clamp for 20mm (Autodesk Fusion 360 design; units mm, degrees)
Autodesk Fusion 360 part; units mm, degrees
note: some values were not read from the file. Set by a fixed rule: which sketch regions a step uses.
sketch "Sketch1" plane through (0, 0, 0) normal (0, 1, 0) x (1, 0, 0)
  line L0 (0, 0) -> (40, 0)
  line L1 (40, 0) -> (40, -16)
  line L2 (40, -16) -> (0, -16)
  line L3 (0, -16) -> (0, 0)
  line L4 (0, -16) -> (40, -16)
  line L5 (40, -16) -> (40, -20)
  line L6 (40, -20) -> (0, -20)
  line L7 (0, -20) -> (0, -16)
  dimension "d1" = 16
  dimension "d2" = 40
  dimension "d3" = 4
  constraint horizontal L0
  constraint vertical L1
  constraint horizontal L2
  constraint vertical L3
  constraint coincident L0.start L3.end
  constraint horizontal L4
  constraint vertical L5
  constraint horizontal L6
  constraint vertical L7
  measures "d1" distance of L0.start L2.end
  measures "d2" distance of L0.start L0.end
  measures "d3" distance of L2.end L6.end
extrude "Extrude1" add sketch "Sketch1" along normal blind 4 makes body 1
extrude "Extrude2" add sketch "Sketch1" against normal blind 8 contours L2 L4 L5 L6 L7 bodies 1
sketch "Sketch2" plane through (0, 0, 0) normal (-1, 0, 0) x (0, 0, 1)
  line L0 (20, -8) -> (20, 4)
  line L1 (20, 4) -> (0, 4)
  line L2 (0, 4) -> (0, 0)
  line L3 (0, 0) -> (16, 0)
  line L4 (16, 0) -> (16, -8)
  line L5 (16, -8) -> (20, -8)
sketch "Sketch3" plane through (0, 0, 20) normal (0, 0, 1) x (1, 0, 0)
  line L0 (40, -8) -> (40, 4)
  line L1 (40, 4) -> (0, 4)
  line L2 (0, 4) -> (0, -8)
  line L3 (0, -8) -> (40, -8)
  line L4 (0, -8) -> (40, -8)
  line L5 (0, 4) -> (0, -8)
  line L6 (0, 0) -> (0, -8)
  line L7 (40, 0) -> (40, -8)
  line L8 (40, -4) -> (0, -4)
  line L9 (40, -4) -> (20, -4)
  line L10 (20, -4) -> (0, -4)
  line L11 (0, -4) -> (10, -4)
  line L12 (40, -4) -> (30, -4)
  line L13 (40, -4) -> (20, -4)
  circle A0 centre (20, -4) radius 3
  circle A1 centre (20, -4) radius 1.5
  circle A2 centre (30, -4) radius 3
  circle A3 centre (30, -4) radius 1.5
  circle A4 centre (10, -4) radius 3
  circle A5 centre (10, -4) radius 1.5
  point P0 (40, 0)
  dimension "d8" = 20
  dimension "d9" = 6
  dimension "d10" = 3
  dimension "d11" = 6
  dimension "d12" = 3
  dimension "d13" = 6
  dimension "d14" = 3
  constraint coincident L2.end L3.start
  constraint coincident L0.start L3.end
  constraint coincident L1.end L2.start
  constraint coincident L6.start origin
  constraint coincident P0 L7.start
  constraint midpoint L7 L8.start
  constraint midpoint L6 L8.end
  constraint midpoint L8 L9.end
  constraint midpoint L10 L11.end
  constraint midpoint L9 L12.end
  constraint coincident L9.end L10.start
  constraint concentric A0 A1
  constraint coincident L12.end A2.centre
  constraint coincident L11.end A4.centre
  measures "d8" distance of L8.start L9.end
  measures "d9" diameter of A0
  measures "d10" diameter of A1
  measures "d11" diameter of A2
  measures "d12" diameter of A3
  measures "d13" diameter of A4
  measures "d14" diameter of A5
extrude "Extrude3" cut sketch "Sketch3" against normal blind 4 contours L8 L9 L12 L13 A3 | L8 L9 L12 L13 A3 bodies 1
extrude "Extrude4" cut sketch "Sketch3" against normal blind 4 contours L8 L9 L10 L13 A1 | L8 L9 L10 L13 A1 bodies 1
extrude "Extrude5" cut sketch "Sketch3" against normal blind 4 contours L8 L10 L11 A5 | L8 L10 L11 A5 bodies 1
extrude "Extrude6" cut sketch "Sketch3" against normal blind 2 contours L8 L9 L12 L13 A2 A3 | L8 L9 L12 L13 A2 A3 | L8 L10 L11 A4 A5 | L8 L10 L11 A4 A5 | L8 L9 L10 L13 A0 A1 | L8 L9 L10 L13 A0 A1 bodies 1
sketch "Sketch4" plane through (0, 0, 0) normal (0, -1, 0) x (1, 0, 0)
  line L0 (40, 16) -> (0, 16)
  line L1 (0, 16) -> (0, 0)
  line L2 (0, 0) -> (40, 0)
  line L3 (40, 0) -> (40, 16)
  line L4 (0, 0) -> (0, 8)
  line L5 (0, 8) -> (40, 8)
  line L6 (0, 8) -> (20, 8)
  line L7 (20, 8) -> (40, 8)
  circle A0 centre (10, 8) radius 3
  circle A1 centre (20, 8) radius 3
  circle A2 centre (30, 8) radius 3
  circle A3 centre (10, 8) radius 1.5
  circle A4 centre (20, 8) radius 1.5
  circle A5 centre (30, 8) radius 1.5
  dimension "d23" = 8
  dimension "d24" = 6
  dimension "d25" = 6
  dimension "d26" = 6
  dimension "d27" = 3
  dimension "d28" = 3
  dimension "d29" = 3
  constraint coincident L1.end L2.start
  constraint midpoint L3 L5.end
  constraint perpendicular L3 L5
  constraint midpoint L5 L6.end
  constraint midpoint L6 A0.centre
  constraint coincident L6.end L7.start
  constraint midpoint L7 A2.centre
  constraint concentric A0 A3
  constraint concentric A2 A5
  measures "d23" distance of L1.end L4.end
  measures "d24" diameter of A0
  measures "d25" diameter of A1
  measures "d26" diameter of A2
  measures "d27" diameter of A3
  measures "d28" diameter of A4
  measures "d29" diameter of A5
extrude "Extrude7" cut sketch "Sketch4" against normal blind 2 contours L5 L7 A2 A5 | L5 L7 A2 A5 | L5 L6 A0 A3 | L5 L6 A0 A3 | L5 L6 L7 A1 A4 | L5 L6 L7 A1 A4 bodies 1
extrude "Extrude8" cut 3 faces at (29.78, 0, 8.964) (19.78, 0, 8.964) (10.5866, 0, 7.6267) along direction (0, 1, 0) blind 30 on bodies 1 bodies 1
mirror "Mirror1" about plane through (0, 0, 0) normal (0, 0, -1) of bodies 1 makes body 2
move_body "Move1" bodies 1 to x (1, 0, 0) y (0, 1, 0) z (0, 0, 1) at (0, 0, -20)
sketch "Sketch5" plane through (0, 0, -4) normal (0, 0, -1) x (-1, 0, 0)
  circle A0 centre (-10, -4) radius 1.5
  circle A1 centre (-20, -4) radius 1.5
  circle A2 centre (-30, -4) radius 1.5
  line L0 (0, 0) -> (-40, 0)
  line L1 (-40, 0) -> (-40, -8)
  line L2 (-40, -8) -> (0, -8)
  line L3 (0, -8) -> (0, 0)
sketch "Sketch6" plane through (0, 0, 0) normal (-1, 0, 0) x (0, 0, 1)
  line L0 (0, -8) -> (0, 4)
  line L1 (0, 4) -> (-20, 4)
  line L2 (-20, 4) -> (-20, 0)
  line L3 (-20, 0) -> (-4, 0)
  line L4 (-4, 0) -> (-4, -8)
  line L5 (-4, -8) -> (0, -8)
  point P0 (-16, 0)
move_body "Move2" bodies 1 to x (1, 0, 0) y (0, 1, 0) z (0, 0, 1) at (0, 0, 4)
combine "Combine1" operation add target body 2 tool bodies 1
equation "d23 = 16 mm / 2"
